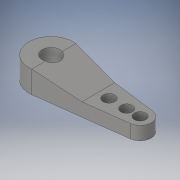
# Autodesk Inventor part: Servo-Arm-20mm
Saved by Autodesk Inventor 2018.2 (Build 222227000, 227)
## iProperties
Created: 2018-02-17
Part Number: Servo-Arm-20mm
Material: Generisch
Document SubType Name: Modeling
Designer: JochenAlt
Density: 1 g/cm^3
Appearance: Vorgabe
Author: JochenAlt
Autodesk Inventor part; units mm, degrees
ref_plane "YZ Plane" through (0, 0, 0) normal (1, 0, 0) x (0, 1, 0)
ref_plane "XZ Plane" through (0, 0, 0) normal (0, 1, 0) x (-1, 0, 0)
ref_plane "XY Plane" through (0, 0, 0) normal (0, 0, 1) x (1, 0, 0)
sketch "Skizze1" plane through (0, 0, 0) normal (0, 0, 1) x (1, 0, 0)
  line L0 (0, 7) -> (0, -7) construction
  line L1 (-10.5, 0) -> (28, 0) construction
  circle A0 centre (0, 0) radius 2
  circle A1 centre (13, 0) radius 1.3257
  circle A2 centre (17, 0) radius 1.3
  circle A3 centre (20, 0) radius 1.3
  arc A4 (20.3125, -2.4804) -> (20.3125, 2.4804) centre (20, 0) ccw
  arc A5 (0.625, 4.9608) -> (0.625, -4.9608) centre (0, 0) ccw
  line L2 (0.625, 4.9608) -> (20.3125, 2.4804)
  line L3 (0.625, -4.9608) -> (20.3125, -2.4804)
  line L4 (0.625, -4.9608) -> (0.625, -1.8998)
  line L5 (0.625, 1.8998) -> (0.625, 4.9608)
  line L6 (0.625, 1.8998) -> (0.625, -1.8998)
  dimension "d0" = 13
  dimension "d1" = 17
  dimension "d2" = 20
  dimension "d3" = 5
  dimension "d4" = 2.6
  dimension "d5" = 4
  dimension "d6" = 10
  constraints: 10 end point, 7 point on circle, 6 centre point, 4 tangent, 3 coincident, 3 point on line, 1 collinear, 1 equal radius, 1 vertical
  measures "d0" distance of A1.centre point (0, 0)
  measures "d1" distance of point (0, 0) A2.centre
  measures "d2" distance of A3.centre point (0, 0)
  measures "d3" diameter of A4
  measures "d4" diameter of A3
  measures "d5" diameter of A0
  measures "d6" diameter of A5
extrude "Extrusion1" add sketch "Skizze1" along normal blind 3
extrude "Extrusion2" add sketch "Skizze1" along normal blind 5 contours L6 A0 | A0 L4 A5 L5 picked at (-0.25, 0)
chamfer "Fase1" distance 10 distance2 2 1 edges at (0.625, 0, 3) measured on face at (4.3081, 0, 3)
extrude "Extrusion3" cut sketch "Skizze1" along normal blind 5 contours A0 L6 | L6 A0
